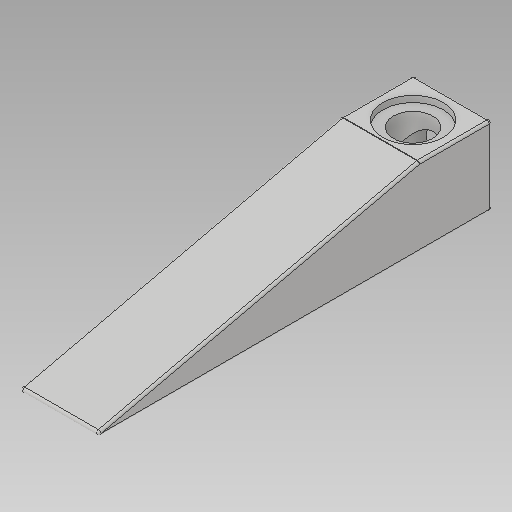
# Autodesk Inventor part: Wedge_base-single
Saved by Autodesk Inventor 2019.3 (Build 233278000, 278)
## iProperties
Created: 2019-02-07
Part Number: Wedge_base-single
Material: Generic
Document SubType Name: Modeling
Designer: Varga Daniel
Density: 1 g/cm^3
Appearance: Default
Author: Varga Daniel
Autodesk Inventor part; units mm, degrees
ref_plane "YZ Plane" through (0, 0, 0) normal (1, 0, 0) x (0, 1, 0)
ref_plane "XZ Plane" through (0, 0, 0) normal (0, 1, 0) x (-1, 0, 0)
ref_plane "XY Plane" through (0, 0, 0) normal (0, 0, 1) x (1, 0, 0)
derived "Connector_pin_base.ipt"
sketch "Pin_base_sketch" plane through (0, 0, 0) normal (0, 0, 1) x (1, 0, 0)
  line L0 (0, 0) -> (23.091816, 0) construction
  line L1 (0, 0) -> (0, 6.219958) construction
  line L2 (0, 3.75) -> (0.55, 3.75)
  line L3 (0.85, 3.45) -> (0.85, 2.4375)
  line L4 (0.85, 2.4375) -> (10.1, 2.4375)
  line L5 (10.1, 2.4375) -> (10.1, 0)
  line L6 (0, 0) -> (0, 3.75)
  line L7 (0, 0) -> (10.1, 0)
  line L8 (9.35, 2.4375) -> (9.35, 2.625)
  line L9 (10.1, 2.4375) -> (10.1, 2.439882)
  arc A0 (10.1, 2.439882) -> (9.910455, 2.731766) centre (9.780488, 2.439882) ccw
  arc A1 (9.910455, 2.731766) -> (9.35, 2.625) centre (9.707071, 2.275) ccw
  line L10 (9.910455, 2.731766) -> (9.910455, -0.007547) construction
  line L11 (8.958404, 2.775) -> (10.385801, 2.775) construction
  arc A2 (0.85, 3.45) -> (0.55, 3.75) centre (0.55, 3.45) ccw
  line L12 (0.85, 2.4375) -> (0.85, 0)
  line L13 (-0.85, 2.4375) -> (-0.85, 0)
  line L14 (-0.85, 3.45) -> (-0.85, 2.4375)
  arc A3 (-0.55, 3.75) -> (-0.85, 3.45) centre (-0.55, 3.45) ccw
  line L15 (0, 3.75) -> (-0.55, 3.75)
  line L16 (0, 0) -> (-23.091816, 0) construction
  line L17 (0, 0) -> (-10.1, 0)
  line L18 (-0.85, 2.4375) -> (-10.1, 2.4375)
  line L19 (-9.35, 2.4375) -> (-9.35, 2.625)
  arc A4 (-9.35, 2.625) -> (-9.910455, 2.731766) centre (-9.707071, 2.275) ccw
  arc A5 (-9.910455, 2.731766) -> (-10.1, 2.439882) centre (-9.780488, 2.439882) ccw
  line L20 (-10.1, 2.4375) -> (-10.1, 2.439882)
  line L21 (-8.958404, 2.775) -> (-10.385801, 2.775) construction
  line L22 (-9.910455, 2.731766) -> (-9.910455, -0.007547) construction
  line L23 (-10.1, 2.4375) -> (-10.1, 0)
  line L24 (9.725, 3.256261) -> (9.725, -1.186806) construction
  dimension "d18" = 7.5
  dimension "d19" = 0.3
  dimension "d52" = 8.5
  dimension "d53" = 10.1
  measures "d18" diameter of L2 L0
  measures "d19" radius of A2
  measures "d52" distance between parallel lines of L19 L14
  measures "d53" distance between parallel lines of L23 L1
derived "Base_part.ipt"
sketch "Beam_sketch" plane through (0, 0, 0) normal (0, 1, 0) x (-1, 0, 0)
  line L0 (5, 0) -> (25, 0)
  line L1 (30, 5) -> (30, 25)
  line L2 (25, 30) -> (5, 30)
  line L3 (0, 25) -> (0, 5)
  line L4 (5, 29) -> (25, 29)
  line L5 (29, 25) -> (29, 5)
  line L6 (25, 1) -> (5, 1)
  line L7 (1, 5) -> (1, 25)
  circle A0 centre (5, 5) radius 2.5
  circle A1 centre (5, 5) radius 3.5
  arc A2 (25, 0) -> (30, 5) centre (25, 5) ccw
  arc A3 (30, 25) -> (25, 30) centre (25, 25) ccw
  arc A4 (5, 30) -> (0, 25) centre (5, 25) ccw
  arc A5 (0, 5) -> (5, 0) centre (5, 5) ccw
  arc A6 (1, 5) -> (5, 1) centre (5, 5) ccw
  arc A7 (5, 29) -> (1, 25) centre (5, 25) ccw
  arc A8 (29, 25) -> (25, 29) centre (25, 25) ccw
  arc A9 (25, 1) -> (29, 5) centre (25, 5) ccw
  line L8 (49.104079, 15) -> (-27.081003, 15) construction
  line L9 (31.147783, 10) -> (-2.487728, 10) construction
  line L10 (-2.860383, 5) -> (35.495034, 5) construction
  line L11 (5, -2.573633) -> (5, 36.752205) construction
  line L12 (15, -1.49775) -> (15, 34.878435) construction
  line L13 (1.535898, 5.5) -> (1, 5.5)
  line L14 (1.535898, 4.5) -> (1.031373, 4.5)
  line L15 (28.968627, 4.5) -> (8.464102, 4.5)
  line L16 (29, 5.5) -> (8.464102, 5.5)
  line L17 (4.5, 1.535898) -> (4.5, 1.031373)
  line L18 (5.5, 1.535898) -> (5.5, 1)
  line L19 (29, 10.5) -> (1, 10.5)
  line L20 (29, 9.5) -> (1, 9.5)
  line L21 (4.5, 28.968627) -> (4.5, 10.5)
  line L22 (4.5, 9.5) -> (4.5, 8.464102)
  line L23 (5.5, 29) -> (5.5, 10.5)
  line L24 (5.5, 9.5) -> (5.5, 8.464102)
  point P0 (0, 0)
  point P1 (30, 30)
  point P2 (0, 30)
  dimension "d1" = 7
  dimension "d2" = 5
  measures "d2" diameter of A0
sketch "Sketch2" plane through (0, 0, 0) normal (1, 0, 0) x (0, 1, 0)
  line L0 (0, 0) -> (10, 0)
  line L1 (10, 0) -> (10, 9.2)
  line L2 (10, 9.2) -> (0.592245, 49.767772)
  line L3 (0, 49.7) -> (0, 0)
  line L4 (0, 47.895032) -> (8.973463, 9.2)
  line L5 (8.973463, 9.2) -> (0, 9.2)
  arc A0 (0.592245, 49.767772) -> (0, 49.7) centre (0.3, 49.7) ccw
  point P0 (0, 52.321627)
  dimension "d3" = 10
  dimension "d5" = 1
  dimension "d6" = 9.2
  dimension "d38" = 0.3
  dimension "d39" = 50
  constraints: 12 end point, 5 point on line, 2 parallel, 2 perpendicular, 2 point on circle, 2 tangent, 1 centre point, 1 horizontal
  measures "d3" distance between parallel lines of L1 L3
  measures "d5" distance between parallel lines of L2 L4
  measures "d6" distance between parallel lines of L5 L0
  measures "d38" radius of A0
extrude "Extrusion1" add sketch "Sketch2" against normal blind 10 contours L3 L5 L4 A0 L2 L1 L0
extrude "Left_wall" add sketch "Sketch2" against normal blind 1 contours L3 L4 L5
sketch "Sketch3" plane through (-10, 0, 0) normal (-1, 0, 0) x (0, 0, 1)
  line L0 (9.2, 8.973463) -> (9.2, 0)
  line L1 (47.895032, 0) -> (9.2, 8.973463)
  line L2 (49.7, 0) -> (0, 0)
  point P0 (50, 0)
extrude "Right_wall" add sketch "Sketch3" against normal blind 1
sketch "Sketch4" plane through (-10, 0, 0) normal (0, -1, 0) x (1, 0, 0)
  line L0 (9, 47.895032) -> (1, 47.895032) construction
  line L1 (9, 9.2) -> (1, 9.2) construction
  line L2 (10, 0) -> (0, 0) construction
  circle A0 centre (5, 5) radius 3.85
  circle A1 centre (5, 5) radius 2.5
  line L3 (10, 49.7) -> (0, 49.7)
  line L4 (0, 0) -> (0, 49.7)
  line L5 (10, 49.7) -> (10, 0)
  line L6 (1, 47.895032) -> (1, 9.2)
  line L7 (9, 9.2) -> (9, 47.895032)
  dimension "d14" = 5
  dimension "d15" = 5
  dimension "d16" = 7.7
  constraints: 2 centre point, 1 coincident
  measures "d14" distance from line of A0.centre L2
  measures "d15" diameter of A1
  measures "d16" diameter of A0
extrude "Extrusion4" cut sketch "Sketch4" against normal through all contours A1
extrude "Extrusion6" cut sketch "Sketch4" against normal blind 0.8
sketch "Sketch6" plane through (0, 10, 9.2) normal (0, 1, 0) x (1, 0, 0)
  circle A0 centre (-5, 4.2) radius 3.85 projected
  circle A1 centre (-5, 4.2) radius 2.5 projected
  point P0 (0, 9.2)
extrude "Extrusion7" cut sketch "Sketch6" against normal blind 0.8
sketch "Sketch10" plane through (0, 0, 0) normal (0, 0, -1) x (-1, 0, 0)
  line L0 (0, 0) -> (0, 10) construction
  line L1 (0, 0) -> (10, 0) construction
  line L2 (10, 10) -> (10, 0) construction
  line L3 (0, 10) -> (10, 10) construction
  circle A0 centre (5, 5) radius 2.5
  circle A1 centre (5, 5) radius 3.85
  dimension "d43" = 5
  dimension "d44" = 7.7
  dimension "d45" = 5
  dimension "d46" = 5
  constraints: 2 centre point, 1 coincident
  measures "d43" diameter of A0
  measures "d44" diameter of A1
  measures "d45" distance from line of A0.centre L2
  measures "d46" distance from line of A0.centre L1
extrude "Extrusion11" cut sketch "Sketch10" against normal up to surface (9.2 mm away) contours A0
extrude "Extrusion12" cut sketch "Sketch10" against normal blind 0.8
fillet "Fillet1" radius 0.3 3 edges at (-5, 10, 0) (-5, 0, 0) (-5, 10, 9.2)
fillet "Left_fillet" radius 0.3 1 edges at (0, 0.2659, 49.9981)
fillet "Right_fillet" radius 0.3 1 edges at (-10, 0.2659, 49.9981)
equation "\"d5\" = Wall_thickness"
equation "\"d6\" = 0.5 * Overall_height + 0.5 * Hole_height"
equation "\"d38\" = Wedge_end_fillet_radius"
equation "\"d39\" = Wedge_length"
equation "\"d9\" = Wall_thickness"
equation "\"d11\" = Wall_thickness"
equation "\"d15\" = d2"
equation "\"d16\" = d18 + Wedge_Pin_collar_diameter_tolerance"
equation "\"d20\" = Wall_thickness"
equation "\"d24\" = -0.5 * Hole_height + 0.5 * Overall_height"
equation "\"d26\" = -0.5 * Hole_height + 0.5 * Overall_height"
equation "\"d43\" = d15"
equation "\"d44\" = d16"
equation "\"d50\" = -0.5 * Hole_height + 0.5 * Overall_height"
equation "\"d40\" = Wedge_fillet_radius"
equation "\"d41\" = Wedge_fillet_radius"
equation "\"d42\" = Wedge_fillet_radius"
equation "\"Wedge_Pin_collar_diameter_tolerance\" = 0.2"
equation "\"Wedge_end_fillet_radius\" = 0.3"
equation "\"Wedge_wall_thickness\" = Wall_thickness"
equation "\"Wedge_fillet_radius\" = 0.3"
equation "\"Wall_thickness\" = 1"
equation "\"Overall_height\" = 10"
equation "\"Hole_height\" = 8.4"
equation "\"Wedge_length\" = 50"
body "Solid1"
